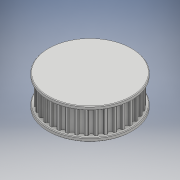
# Autodesk Inventor part: Gear 35 Teeth
Saved by Autodesk Inventor 2018 (Build 220112000, 112)
## iProperties
Created: 2018-05-29
Part Number: Gear 35 Teeth
Material: Generic
Document SubType Name: Modeling
Designer: P301319
Density: 1 g/cm^3
Appearance: Default
Author: P301319
Autodesk Inventor part; units mm, degrees
ref_plane "YZ Plane" through (0, 0, 0) normal (1, 0, 0) x (0, 1, 0)
ref_plane "XZ Plane" through (0, 0, 0) normal (0, 1, 0) x (-1, 0, 0)
ref_plane "XY Plane" through (0, 0, 0) normal (0, 0, 1) x (1, 0, 0)
sketch "Tooth" plane through (0, 0, 0) normal (0, 0, 1) x (1, 0, 0)
  arc A0 (0, 16.7113) -> (-1.498, 16.644) centre (0, 0) ccw construction
  line L0 (0, 0) -> (0, 16.7113) construction
  line L1 (0, 0) -> (-1.498, 16.644) construction
  circle A1 centre (0, 0) radius 15.5713 construction
  arc A2 (-0.773, 16.0678) -> (0, 15.5713) centre (0, 16.4213) ccw
  arc A3 (0.6099, 16.7001) -> (0, 16.7113) centre (0, 0) ccw construction
  arc A4 (-0.8918, 16.4611) -> (-0.773, 16.0678) centre (0.6099, 16.7001) ccw
  arc A5 (-1.156, 16.6712) -> (-1.498, 16.644) centre (0, 0) ccw
  arc A6 (-0.8918, 16.4611) -> (-1.156, 16.6712) centre (-1.1387, 16.4218) ccw
  arc A7 (0, 15.5713) -> (0.773, 16.0678) centre (0, 16.4213) ccw
  arc A8 (0.773, 16.0678) -> (0.8918, 16.4611) centre (-0.6099, 16.7001) ccw
  arc A9 (1.498, 16.644) -> (1.156, 16.6712) centre (0, 0) ccw
  arc A10 (1.156, 16.6712) -> (0.8918, 16.4611) centre (1.1387, 16.4218) ccw
  arc A11 (1.6773, 18.6359) -> (-1.6773, 18.6359) centre (0, 0) ccw
  line L2 (1.498, 16.644) -> (1.6773, 18.6359)
  line L3 (-1.498, 16.644) -> (-1.6773, 18.6359)
  dimension "d2" = 16.7113
  dimension "d3" = 1.5
  dimension "d4" = 1.14
  dimension "d5" = 0.85
  dimension "d6" = 0.61
  dimension "d7" = 0.25
  dimension "d8" = 2
  constraints: 22 point on circle, 11 centre point, 8 end point, 6 symmetric about line, 5 coincident, 4 line through centre, 3 tangent, 2 vertical alignment, 1 concentric, 1 vertical, 7 other
  measures "d2" radius of A0
  measures "d5" radius of A2
  measures "d7" radius of A6
  measures "d8" radial gap between concentric circles of A11 A0
sketch "Sketch2" plane through (0, 0, 0) normal (0, 0, 1) x (1, 0, 0)
  circle A0 centre (0, 0) radius 16.7113
  arc A1 (-1.156, 16.6712) -> (-1.498, 16.644) centre (0, 0) ccw projected
  arc A2 (1.498, 16.644) -> (1.156, 16.6712) centre (0, 0) ccw projected
  dimension "d9" = 16.7113
  constraints: 1 centre point, 1 coincident
  measures "d9" radius of A0
extrude "Gear Solid Extrusion" add sketch "Sketch2" along normal blind 10
extrude "Tooth Cut-Out Extrusion" cut sketch "Tooth" along normal blind 10
pattern_circular "Teeth Array" count 35 over 360 about axis through (0, 0, 0) along (0, 0, 1) of "Tooth Cut-Out Extrusion"
sketch "Sketch3" plane through (0, 0, 10) normal (0, 0, 1) x (1, 0, 0)
  circle A0 centre (0, 0) radius 17.7113
  dimension "d17" = 17.7113
  constraints: 1 centre point, 1 coincident
  measures "d17" radius of A0
extrude "Flange Extrusion Front" add sketch "Sketch3" along normal blind 1.5
sketch "Sketch4" plane through (0, 0, 0) normal (0, 0, -1) x (-1, 0, 0)
  circle A0 centre (0, 0) radius 17.7113
  dimension "d20" = 17.7113
  constraints: 1 centre point, 1 coincident
  measures "d20" radius of A0
extrude "Flange Extrusion Back" add sketch "Sketch4" along normal blind 1.5
fillet "Flange Fillet" radius 0.25 4 edges at (17.7113, 0, -1.5) (-17.7113, 0, 11.5) (-17.7113, 0, 10) (17.7113, 0, 0)
equation "\"d3\" = HalfPitch"
equation "\"d12\" = ToothWidth"
equation "\"d21\" = FlangeWidth"
equation "\"HalfPitch\" = 1.5"
equation "\"ToothWidth\" = 10"
equation "\"FlangeWidth\" = 1.5"
body "Solid1"
